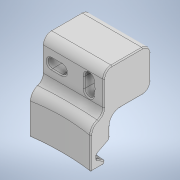
# Autodesk Inventor part: hoop_holder_158mm
Saved by Autodesk Inventor 2022 (Build 260153000, 153)
## iProperties
Created: 2022-02-22
Part Number: hoop_holder_158mm
Material: Generic
Document SubType Name: Modeling
Designer: Frey
Density: 1 g/cm^3
Appearance: Default
Author: Frey
Autodesk Inventor part; units mm, degrees
ref_plane "YZ Plane" through (0, 0, 0) normal (1, 0, 0) x (0, 1, 0)
ref_plane "XZ Plane" through (0, 0, 0) normal (0, 1, 0) x (-1, 0, 0)
ref_plane "XY Plane" through (0, 0, 0) normal (0, 0, 1) x (1, 0, 0)
sketch "Sketch2" plane through (0, 0, 0) normal (0, 1, 0) x (-1, 0, 0)
  circle A0 centre (0, 0) radius 114.3 construction
  arc A1 (-15, -119.7139) -> (15, -119.7139) centre (0, 0) ccw
  arc A2 (15, -110.2846) -> (-15, -110.2846) centre (0, 0) ccw construction
  line L0 (15, -110.2846) -> (15, -119.7139)
  line L1 (-15, -110.2846) -> (-15, -119.7139)
  arc A3 (15, -119.7139) -> (-15, -119.7139) centre (0, 0) ccw construction
  arc A4 (-15, -110.2846) -> (15, -110.2846) centre (0, 0) ccw
  dimension "d1" = 228.6
  dimension "d2" = 241.3
  dimension "d3" = 222.6
  dimension "d4" = 30
  constraints: 8 point on circle, 5 centre point, 4 end point, 3 coincident, 2 horizontal alignment, 1 parallel, 1 vertical
  measures "d1" diameter of A0
  measures "d2" diameter of A1
  measures "d3" diameter of A2
  measures "d4" distance between parallel lines of L1 L0
extrude "Extrusion1" add sketch "Sketch2" along normal blind 20
sketch "Sketch3" plane through (0, 0, 0) normal (1, 0, 0) x (0, 1, 0)
  line L0 (5.7297, -114.3) -> (4.3114, -114.3)
  line L1 (6.1757, -114.5738) -> (9.5868, -121.3)
  line L2 (9.5868, -121.3) -> (-0.4132, -121.3)
  line L3 (-0.4132, -121.3) -> (3.8895, -114.5318)
  line L4 (6.0368, -114.3) -> (-0.4132, -121.3) construction
  line L5 (4.0368, -114.3) -> (9.5868, -121.3) construction
  line L6 (-2.2005, 0) -> (10.7495, 0) projected
  line L7 (0, -120.65) -> (0, -119.7139) projected
  arc A0 (6.1757, -114.5738) -> (5.7297, -114.3) centre (5.7297, -114.8) ccw
  arc A1 (4.3114, -114.3) -> (3.8895, -114.5318) centre (4.3114, -114.8) ccw
  point P0 (0, 0)
  point P1 (4.9618, -115.4667)
  dimension "d7" = 2
  dimension "d8" = 10
  dimension "d9" = 114.3
  dimension "d10" = 7
  dimension "d11" = 4.625
  dimension "d13" = 0.5
  constraints: 12 end point, 7 point on line, 4 point on circle, 4 tangent, 2 centre point, 2 horizontal, 1 equal radius
  measures "d7" distance of L4.start L5.start
  measures "d8" distance of L1.end L2.end
  measures "d9" vertical distance of point (0, 0) L5.start
  measures "d10" distance between parallel lines of L2 L0
  measures "d11" horizontal distance of point (4.962, -115.467) L1.end
  measures "d13" radius of A0
revolve "Revolution1" cut sketch "Sketch3" angle 360 about axis through (0, -10, 0) along (0, 1, 0)
fillet "Fillet1" radius 2 2 edges at (7.5145, 9.2571, -120.4158) (-7.5146, 9.2571, -120.4158)
fillet "Fillet2" radius 1 1 edges at (0, 0, -120.65)
sketch "Sketch4" plane through (0, 20, 0) normal (0, 1, 0) x (1, 0, 0)
  line L0 (-15, 119.7139) -> (-15, 110.2846) projected
  line L1 (15, 110.2846) -> (15, 119.7139) projected
  line L2 (-15, 116.7139) -> (15, 116.7139)
  line L3 (15, 110.2846) -> (15, 116.2492) projected
  line L4 (15, 119.7139) -> (-15, 119.7139)
  arc A0 (15, 110.2846) -> (-15, 110.2846) centre (0, 0) ccw projected
  point P0 (15, 116.7139)
  dimension "d16" = 3
  constraints: 4 end point, 3 point on line, 2 perpendicular
  measures "d16" distance between parallel lines of L4 L2
extrude "Extrusion2" add sketch "Sketch4" along normal blind 20 contours L4 L1 L2 L0
fillet "Fillet3" radius 4 1 edges at (0, 20, -116.7139)
fillet "Fillet4" radius 5 1 edges at (0, 20, -111.3)
sketch "Sketch7" plane through (15, 20, -119.7139) normal (0, 0, -1) x (-1, 0, 0)
  line L0 (30, 0) -> (0, 0) projected
  line L1 (30, 0) -> (30, 20) projected
  line L2 (0, 20) -> (30, 20) projected
  line L3 (0, 0) -> (0, 20) projected
  point P0 (15, -20)
extrude "Extrusion4" add sketch "Sketch7" along normal blind 20
sketch "Sketch8" plane through (-15, 40, -116.7139) normal (0, 0, 1) x (1, 0, 0)
  line L0 (4.5, -10) -> (9.5, -10) construction
  line L1 (4.5, -12.25) -> (9.5, -12.25)
  line L2 (9.5, -7.75) -> (4.5, -7.75)
  arc A0 (4.5, -7.75) -> (4.5, -12.25) centre (4.5, -10) ccw
  arc A1 (9.5, -12.25) -> (9.5, -7.75) centre (9.5, -10) ccw
  arc A2 (22.7162, -13) -> (22.7162, -7) centre (7, -10) ccw construction
  arc A3 (24.9263, -13.4219) -> (24.9263, -6.5781) centre (7, -10) ccw
  arc A4 (20.5061, -12.5781) -> (20.5061, -7.4219) centre (7, -10) ccw
  arc A5 (20.5061, -12.5781) -> (24.9263, -13.4219) centre (22.7162, -13) ccw
  arc A6 (24.9263, -6.5781) -> (20.5061, -7.4219) centre (22.7162, -7) ccw
  line L3 (30, 0) -> (30, -20) projected
  line L4 (0, -20) -> (0, 0) projected
  line L5 (0, 0) -> (30, 0) projected
  point P0 (15, -40)
  dimension "d67" = 16
  dimension "d68" = 5
  dimension "d69" = 6
  dimension "d70" = 4.5
  dimension "d71" = 4.5
  dimension "d72" = 30
  dimension "d73" = 7
  dimension "d74" = 10
  constraints: 14 point on circle, 8 end point, 8 tangent, 7 centre point, 1 coincident, 1 horizontal, 1 midpoint, 1 parallel, 1 vertical alignment
  measures "d67" radius of A2
  measures "d68" distance of L0.end L0.start
  measures "d69" distance of A2.start A2.end
  measures "d70" distance between parallel lines of L1 L2
  measures "d71" radial gap between concentric circles of A3 A4
  measures "d72" distance between parallel lines of L3 L4
  measures "d73" distance from line of point (7, -10) L4
  measures "d74" distance between parallel lines of L0 L5
extrude "Extrusion5" cut sketch "Sketch8" against normal up to surface (23 mm away)
fillet "Fillet9" radius 5 1 edges at (0, 20, -120.65)
fillet "Fillet11" radius 0.5 51 edges at (15, 30, -139.7139) (15, 20, -132.2327) (15, 18.5417, -121.196) (15, 12.7427, -119.7139) (15, 9.4387, -119.4159) (15, 7.425, -116.0721) (15, 5.9915, -113.3861) (15, 5.0206, -113.3115) (15, 4.0706, -113.3738) (15, 2.8739, -115.1565) (15, 0.7197, -117.217) (15, 0, -113.2669) (15, 32, -116.7139) (15, 21.6174, -115.9269) (15, 18.3646, -111.289) (15, 7.6826, -110.2846) (15, 40, -128.2139) (-15, 30, -139.7139) (-15, 20, -132.2327) (-15, 18.5417, -121.196) (-15, 12.7427, -119.7139) (-15, 9.4387, -119.4159) (-15, 7.425, -116.0721) (-15, 5.9915, -113.3861) (-15, 5.0206, -113.3115) (-15, 4.0706, -113.3738) (-15, 2.8739, -115.1565) (-15, 0.7197, -117.217) (-15, 0, -113.2669) (-15, 32, -116.7139) (-15, 21.6174, -115.9269) (-15, 18.3646, -111.289) (-15, 7.6826, -110.2846) (-15, 40, -128.2139) (-3.25, 30, -116.7139) (-8, 27.75, -116.7139) (-12.75, 30, -116.7139) (-8, 32.25, -116.7139) (10.25, 30, -116.7139) (7.2944, 24.7899, -116.7139) (5.75, 30, -116.7139) (7.2944, 35.2101, -116.7139) (5.75, 30, -139.7139) (7.2944, 24.7899, -139.7139) (10.25, 30, -139.7139) (7.2944, 35.2101, -139.7139) (-12.75, 30, -139.7139) (-8, 27.75, -139.7139) (-3.25, 30, -139.7139) (-8, 32.25, -139.7139) (0, 0, -111.3)
fillet "Fillet12" radius 4 3 edges at (14.8536, 39.8536, -116.8604) (-14.8536, 39.8536, -116.8604) (0, 40, -116.7139)
fillet "Fillet13" radius 4 66 edges at (14.8743, 15, -119.6034) (15, 18.8908, -120.8962) (14.8743, 10.4854, -119.6034) (15, 12.7427, -119.2718) (14.8631, 8.8386, -118.595) (15, 9.6938, -119.0444) (14.8636, 6.3126, -113.5744) (15, 7.871, -115.9079) (14.8754, 5.7297, -113.2027) (15, 6.2701, -113.033) (14.8754, 4.3114, -113.2027) (15, 5.0206, -112.8725) (14.8654, 3.7589, -113.5177) (15, 3.8149, -113.006) (14.8651, 1.7132, -116.7617) (15, 2.4558, -114.944) (14.8536, 0.1464, -116.3127) (15, 0.8107, -116.781) (14.8536, 0.1464, -110.8557) (15, 0.5, -113.5842) (14.8298, 0.5, -110.4799) (14.8298, 15.3886, -110.4799) (15, 7.9443, -110.8557) (15, 18.0577, -111.7369) (14.8536, 20.0413, -113.9476) (15, 21.3331, -116.3385) (14.8536, 24, -116.8604) (14.8536, 36, -116.8604) (15, 30, -117.2139) (-15, 18.8908, -120.8962) (-15, 12.7427, -119.2718) (-15, 9.6938, -119.0444) (-15, 7.871, -115.9079) (-15, 6.2701, -113.033) (-15, 5.0206, -112.8725) (-15, 3.8149, -113.006) (-15, 2.4558, -114.944) (-15, 0.8107, -116.781) (-15, 0.5, -113.5842) (-15, 7.9443, -110.8557) (-15, 18.0577, -111.7369) (-15, 21.3331, -116.3385) (-15, 30, -117.2139) (-14.8743, 15, -119.6034) (-14.8743, 10.4854, -119.6034) (-14.8631, 8.8386, -118.595) (-14.8636, 6.3126, -113.5744) (-14.8754, 5.7297, -113.2027) (-14.8754, 4.3114, -113.2027) (-14.8654, 3.7589, -113.5177) (-14.8651, 1.7132, -116.7617) (-14.8536, 0.1464, -116.3127) (-14.8536, 0.1464, -110.8557) (-14.8298, 0.5, -110.4799) (-14.8298, 15.3886, -110.4799) (-14.8536, 20.0413, -113.9476) (-14.8536, 24, -116.8604) (-14.8536, 36, -116.8604) (0, 40, -139.7139) (-14.5, 20, -132.2622) (-14.8536, 20.1464, -139.5675) (-14.5, 30, -139.7139) (14.5, 20, -132.2622) (14.5, 30, -139.7139) (14.8536, 20.1464, -139.5675) (0, 20, -139.7139)
body "Solid1"
